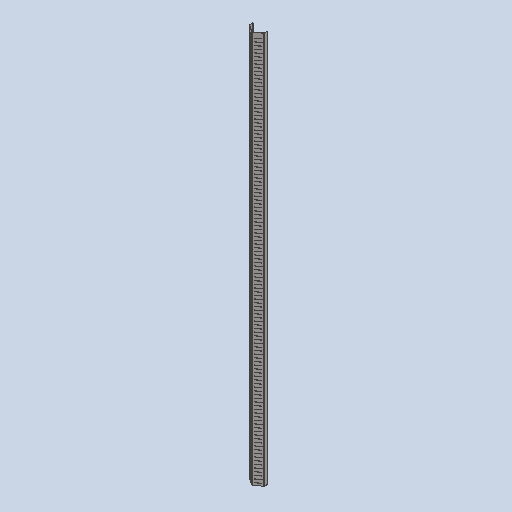
# Autodesk Inventor part: NDV-3102 Branch roof 01
Saved by Autodesk Inventor 2026.2 (Build 302298000, 298)
## iProperties
Created: 2026-10-05
Part Number: NDV-3102 Branch roof 01
Material: Stainless Steel
Document SubType Name: Sheet Metal
Designer: admin
Density: 8 g/cm^3
Sheet Metal Rule: Default_mm
Appearance: Semi-Polished
Mass: 486.9 g
Surface Area: 1600.56 cm^2
Volume: 60.8626 cm^3
Stock Number: Крышка луча 1
Flat Pattern Width: 6.9707 cm
Flat Pattern Length: 111 cm
Flat Pattern Area: 773.748 cm^2
Sheet Metal Width: 69,707 mm
Sheet Metal Length: 1110,000 mm
Sheet Metal Area: 77374,806 mm^2
Author: admin
Autodesk Inventor part; units mm, degrees
ref_plane "YZ Plane" through (0, 0, 0) normal (1, 0, 0) x (0, 1, 0)
ref_plane "XZ Plane" through (0, 0, 0) normal (0, 1, 0) x (-1, 0, 0)
ref_plane "XY Plane" through (0, 0, 0) normal (0, 0, 1) x (1, 0, 0)
derived "NDV-0010 Parameters 01.ipt"
sketch "sk_roof_profile" plane through (0, 0, 0) normal (0, 1, 0) x (-1, 0, 0)
  line L0 (-20.9563, 0) -> (-20.9563, 10)
  line L1 (-20.9563, 10) -> (0, 25)
  line L2 (0, 25) -> (21.0437, 10.1228)
  line L3 (21.0437, 10.1228) -> (21.0437, 0)
  line L4 (-20.9563, 0) -> (21.0437, 0) construction
  line L5 (0, 0) -> (0, 25) construction
  dimension "d1" = 42
  dimension "d2" = 10
  dimension "d3" = 15
  dimension "d4" = 0
  measures "d1" distance of L0.start L3.end
  measures "d2" distance of L0.start L0.end
  measures "d3" vertical distance of L0.end L1.end
  measures "d4" vertical distance of L5.start L0.start
contour flange "Roof_body" sketch "sk_roof_profile" thickness 0.8 bend radius 0.8 width 1110 along (0, 1, 0) mid plane no both sides no wall seen from (20.9563, 0, 5) lies toward (-1, 0, 0) curves L0 L1 L2 L3
bend "Bend1"
corner "Corner1"
sketch "sk_slots" plane through (0.9255, 0, 24.3375) normal (0.5820395, 0, 0.8131605) x (0.8131605, 0, -0.5820395)
  line L0 (0, 0) -> (0, 1110) projected
  line L1 (23.8109, 0) -> (0, 0) projected
  line L2 (5, 6.5) -> (20, 6.5)
  line L3 (20, 6.5) -> (20, 6.9)
  line L4 (20, 6.9) -> (5, 6.9)
  line L5 (5, 6.9) -> (5, 6.5)
  dimension "d16" = 5
  dimension "d17" = 6.5
  dimension "d18" = 15
  dimension "d19" = 0.4
  constraints: 8 end point, 3 perpendicular, 1 parallel
  measures "d16" distance from line of L0 L2.start
  measures "d17" distance from line of L1 L2.start
  measures "d18" distance from line of L5 L2.end
  measures "d19" distance from line of L2 L4.end
extrude "Slot" cut sketch "sk_slots" against normal blind 0.8
pattern_linear "Slot_pattern" count 122 spacing 9 along (0, 1, 0) of "Slot"
sketch "sk_Slot_L" plane through (-20.3673, 0, 10.601) normal (-0.5772748, 0, 0.81655) x (0.81655, 0, 0.5772748)
  line L0 (23.805, 0) -> (23.805, 1110) projected
  line L1 (23.805, 0) -> (0, 0) projected
  line L2 (18.805, 6.5) -> (3.805, 6.5)
  line L3 (3.805, 6.5) -> (3.805, 6.9)
  line L4 (3.805, 6.9) -> (18.805, 6.9)
  line L5 (18.805, 6.9) -> (18.805, 6.5)
  dimension "d25" = 5
  dimension "d26" = 6.5
  dimension "d27" = 15
  dimension "d28" = 0.4
  constraints: 8 end point, 3 perpendicular, 1 parallel
  measures "d25" distance from line of L0 L2.start
  measures "d26" distance from line of L1 L2.start
  measures "d27" distance from line of L5 L2.end
  measures "d28" distance from line of L2 L4.end
extrude "Slot_L" cut sketch "sk_Slot_L" against normal blind 0.8
pattern_linear "Slot_L_pattern" count 122 spacing 9 along (0, 1, 0) of "Slot_L"
equation "\"d1\" = Roof_w + 2 * Roof_thickness"
equation "\"d2\" = Roof_skirt"
equation "\"d3\" = Roof_rise"
equation "\"d16\" = Slot_ridge_offset"
equation "\"d17\" = 0.5 * Slot_end_offset"
equation "\"d18\" = 0.5 * Slot_length"
equation "\"d19\" = Slot_gap"
equation "\"d25\" = Slot_ridge_offset"
equation "\"d26\" = 0.5 * Slot_end_offset"
equation "\"d27\" = 0.5 * Slot_length"
equation "\"d28\" = Slot_gap"
equation "\"d24\" = Slot_step"
equation "\"d33\" = Slot_step"
equation "\"d5\" = Thickness"
equation "\"d6\" = Thickness"
equation "\"d7\" = 0.5 * Thickness"
equation "\"d8\" = 2 * Thickness"
equation "\"d9\" = Thickness"
equation "\"d10\" = Roof_length_1"
equation "\"d11\" = Thickness"
equation "\"d13\" = 4 * Thickness"
equation "\"d14\" = Roof_thickness"
equation "\"d15\" = JacobiRadiusSize"
equation "\"Thickness\" = Roof_thickness"
equation "\"BendRadius\" = Thickness"
equation "\"BendReliefWidth\" = Thickness"
equation "\"BendReliefDepth\" = 0.5 * Thickness"
equation "\"CornerReliefSize\" = 4 * Thickness"
equation "\"MinimumRemnant\" = 2 * Thickness"
equation "\"TransitionRadius\" = BendRadius"
equation "\"JacobiRadiusSize\" = BendRadius"
equation "\"GapSize\" = Thickness"
equation "\"Roof_w\" = Small_ways_cross + Roof_gap"
equation "\"Slot_ridge_offset\" = 5"
equation "\"Roof_thickness\" = 0.8"
equation "\"Roof_skirt\" = 10"
equation "\"Roof_rise\" = 15"
equation "\"Slot_end_offset\" = 13"
equation "\"Slot_length\" = 30"
equation "\"Slot_gap\" = 0.4"
equation "\"Slot_step\" = 9"
equation "\"Roof_length_1\" = 1110"
equation "\"Small_ways_cross\" = 40"
equation "\"Roof_gap\" = 0.4"
body "Solid1"
